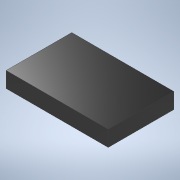
# Autodesk Inventor part: battery_handler
Saved by Autodesk Inventor 2020 (Build 240168000, 168)
## iProperties
Created: 2021-05-30
Part Number: battery_handler
Material: PPS Plastic
Document SubType Name: Modeling
Designer: hasht
Density: 1.637 g/cm^3
Appearance: Glossy - Black
Author: hasht
Autodesk Inventor part; units mm, degrees
ref_plane "YZ Plane" through (0, 0, 0) normal (1, 0, 0) x (0, 1, 0)
ref_plane "XZ Plane" through (0, 0, 0) normal (0, 1, 0) x (-1, 0, 0)
ref_plane "XY Plane" through (0, 0, 0) normal (0, 0, 1) x (1, 0, 0)
sketch "Sketch1" plane through (0, 0, 0) normal (0, 1, 0) x (-1, 0, 0)
  line L0 (0, 0) -> (24.892, 0)
  line L1 (24.892, 0) -> (24.892, -16.002)
  line L2 (24.892, -16.002) -> (0, -16.002)
  line L3 (0, -16.002) -> (0, 0)
  dimension "d0" = 24.892
  dimension "d1" = 16.002
  constraints: 8 end point, 2 parallel, 1 horizontal, 1 perpendicular
  measures "d0" distance of L1.end L2.end
  measures "d1" distance of L0.end L1.end
extrude "Extrusion1" add sketch "Sketch1" along normal blind 3.81
body "Solid1"
